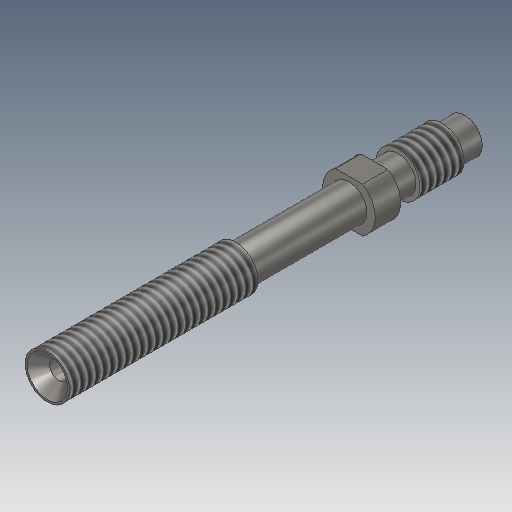
# Autodesk Inventor part: feeder tube
Saved by Autodesk Inventor 2019 (Build 230136000, 136)
## iProperties
Created: 2018-11-13
Part Number: feeder tube
Material: Stainless Steel
Document SubType Name: Modeling
Designer: LillaHunden
Density: 8 g/cm^3
Appearance: Semi-Polished
Mass: 8.7671 g
Surface Area: 14.8668 cm^2
Volume: 1.09589 cm^3
Author: LillaHunden
Autodesk Inventor part; units mm, degrees
ref_plane "YZ Plane" through (0, 0, 0) normal (1, 0, 0) x (0, 1, 0)
ref_plane "XZ Plane" through (0, 0, 0) normal (0, 1, 0) x (-1, 0, 0)
ref_plane "XY Plane" through (0, 0, 0) normal (0, 0, 1) x (1, 0, 0)
sketch "Sketch1" plane through (0, 0, 0) normal (0, 0, 1) x (1, 0, 0)
  circle A0 centre (0, 0) radius 2.365
  dimension "d0" = 4.73
  constraints: 1 centre point, 1 coincident
  measures "d0" diameter of A0
extrude "Extrusion1" add sketch "Sketch1" along normal blind 3
sketch "Sketch2" plane through (0, 0, 3) normal (0, 0, 1) x (1, 0, 0)
  circle A0 centre (0, 0) radius 2.94
  dimension "d3" = 5.88
  constraints: 1 centre point, 1 coincident
  measures "d3" diameter of A0
extrude "Extrusion2" add sketch "Sketch2" along normal blind 5.9
thread "Thread1" size "M6x1" class "6g" standard "ANSI Metric M Profile" full length
sketch "Sketch3" plane through (0, 0, 8.9) normal (0, 0, 1) x (1, 0, 0)
  circle A0 centre (0, 0) radius 2.94 projected
  circle A1 centre (0, 0) radius 2.395
  dimension "d8" = 4.79
  constraints: 1 centre point, 1 coincident
  measures "d8" diameter of A1
extrude "Extrusion3" add sketch "Sketch3" along normal blind 3.15 contours A1
sketch "Sketch4" plane through (0, 0, 12.05) normal (0, 0, 1) x (1, 0, 0)
  circle A0 centre (0, 0) radius 3.5
  dimension "d11" = 7
  constraints: 1 centre point, 1 coincident
  measures "d11" diameter of A0
extrude "Extrusion4" add sketch "Sketch4" along normal blind 3.4
sketch "Sketch5" plane through (0, 0, 15.45) normal (0, 0, 1) x (1, 0, 0)
  line L0 (-1.8028, -3) -> (1.8028, -3)
  line L1 (9.1237, -3) -> (9.1237, 3)
  line L2 (1.8028, 3) -> (-1.8028, 3)
  line L3 (-9.1237, 3) -> (-9.1237, -3)
  line L4 (-9.1237, -3) -> (9.1237, 3) construction
  line L5 (9.1237, -3) -> (-9.1237, 3) construction
  circle A0 centre (0, 0) radius 3.5 projected
  dimension "d14" = 6
  constraints: 12 end point, 4 point on circle, 2 midpoint, 2 parallel, 1 horizontal, 1 perpendicular
  measures "d14" distance of L1.end L1.start
extrude "Extrusion5" cut sketch "Sketch5" against normal blind 3.4 contours L0 A0 | A0 L2
sketch "Sketch6" plane through (0, 0, 15.45) normal (0, 0, 1) x (1, 0, 0)
  circle A0 centre (0, 0) radius 2.4
  dimension "d17" = 4.8
  constraints: 1 centre point, 1 coincident
  measures "d17" diameter of A0
extrude "Extrusion6" add sketch "Sketch6" along normal blind 15.13
sketch "Sketch7" plane through (0, 0, 30.58) normal (0, 0, 1) x (1, 0, 0)
  circle A0 centre (0, 0) radius 2.965
  dimension "d20" = 5.93
  constraints: 1 centre point, 1 coincident
  measures "d20" diameter of A0
extrude "Extrusion7" add sketch "Sketch7" along normal blind 25.17
thread "Thread2" size "M6x1" class "6g" standard "ANSI Metric M Profile" full length
sketch "Sketch8" plane through (0, 0, 55.75) normal (0, 0, 1) x (1, 0, 0)
  circle A0 centre (0, 0) radius 1.2
  dimension "d25" = 2.4
  constraints: 1 centre point, 1 coincident
  measures "d25" diameter of A0
extrude "Extrusion8" cut sketch "Sketch8" against normal through all
chamfer "Chamfer1" distance 1.5 angle 45 1 edges at (-1.2, 0, 55.75)
chamfer "Chamfer2" distance 0.5 angle 45 1 edges at (-1.2, 0, 0)
body "Solid1"
